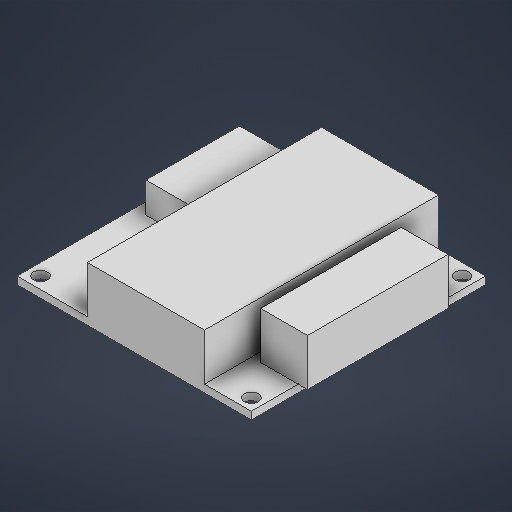
# Autodesk Inventor part: motor_driver
Saved by Autodesk Inventor 2026.2 (Build 302298000, 298)
## iProperties
Created: 2026-03-16
Part Number: motor_driver
Material: Generic
Document SubType Name: Modeling
Designer: User
Density: 1 g/cm^3
Appearance: Default
Author: User
Autodesk Inventor part; units mm, degrees
ref_plane "YZ Plane" through (0, 0, 0) normal (1, 0, 0) x (0, 1, 0)
ref_plane "XZ Plane" through (0, 0, 0) normal (0, 1, 0) x (-1, 0, 0)
ref_plane "XY Plane" through (0, 0, 0) normal (0, 0, 1) x (1, 0, 0)
sketch "Sketch1" plane through (0, 0, 0) normal (0, 1, 0) x (-1, 0, 0)
  line L0 (0, 0) -> (50, 0)
  line L1 (50, 0) -> (50, -50)
  line L2 (50, -50) -> (0, -50)
  line L3 (0, -50) -> (0, 0)
  circle A0 centre (47.5, -2.5) radius 1.5
  circle A1 centre (47.5, -47.5) radius 1.5
  circle A2 centre (2.5, -2.5) radius 1.5
  circle A3 centre (2.5, -47.5) radius 1.5
  dimension "d0" = 50
  dimension "d1" = 50
  dimension "d2" = 3
  dimension "d3" = 3
  dimension "d4" = 3
  dimension "d5" = 3
  dimension "d6" = 2.5
  dimension "d7" = 45
  dimension "d8" = 2.5
  dimension "d9" = 2.5
  dimension "d10" = 2.5
  dimension "d11" = 45
  dimension "d12" = 45
  dimension "d13" = 45
  constraints: 8 end point, 4 centre point, 2 parallel, 1 horizontal, 1 perpendicular
  measures "d0" distance of L1.end L2.end
  measures "d1" distance of L0.end L1.end
  measures "d2" diameter of A0
  measures "d3" diameter of A1
  measures "d4" diameter of A2
  measures "d5" diameter of A3
  measures "d6" distance from line of L1 A0.centre
  measures "d7" distance of A0.centre A2.centre
  measures "d8" distance from line of L0 A0.centre
  measures "d9" distance from line of L1 A1.centre
  measures "d10" distance from line of L0 A2.centre
  measures "d11" distance of A0.centre A1.centre
  measures "d12" distance of A3.centre A1.centre
  measures "d13" distance of A2.centre A3.centre
extrude "Extrusion1" add sketch "Sketch1" along normal blind 1.6
sketch "Sketch2" plane through (0, 1.6, 0) normal (0, 1, 0) x (1, 0, 0)
  line L0 (-10, 0) -> (-35, 0)
  line L1 (-35, 0) -> (-35, 50)
  line L2 (-35, 50) -> (-10, 50)
  line L3 (-10, 50) -> (-10, 0)
  line L4 (-50, 0) -> (0, 0) projected
  line L5 (0, 0) -> (0, 50) projected
  line L6 (2, 10) -> (-8, 10)
  line L7 (-8, 10) -> (-8, 40)
  line L8 (-8, 40) -> (2, 40)
  line L9 (2, 40) -> (2, 10)
  line L10 (-47.5, 45) -> (-38.5, 45)
  line L11 (-38.5, 45) -> (-38.5, 25)
  line L12 (-38.5, 25) -> (-47.5, 25)
  line L13 (-47.5, 25) -> (-47.5, 45)
  line L14 (-50, 50) -> (-50, 0) projected
  line L15 (0, 50) -> (-50, 50) projected
  point P0 (0, 40)
  point P1 (0, 10)
  dimension "d16" = 25
  dimension "d17" = 50
  dimension "d19" = 10
  dimension "d20" = 10
  dimension "d21" = 30
  dimension "d22" = 10
  dimension "d23" = 2
  dimension "d26" = 9
  dimension "d27" = 20
  dimension "d28" = 2.5
  dimension "d29" = 5
  constraints: 24 end point, 6 parallel, 3 horizontal, 3 perpendicular, 1 collinear
  measures "d16" distance of L1.end L2.end
  measures "d17" distance of L0.end L1.end
  measures "d19" distance between parallel lines of L5 L3
  measures "d20" distance of L7.end L8.end
  measures "d21" distance of L6.end L7.end
  measures "d22" distance between parallel lines of L4 L6
  measures "d23" distance between parallel lines of L3 L7
  measures "d26" distance of L11.end L12.end
  measures "d27" distance of L10.end L11.end
  measures "d28" distance between parallel lines of L14 L13
  measures "d29" distance between parallel lines of L10 L15
extrude "Extrusion2" add sketch "Sketch2" along normal blind 10 contours L0 L1 L2 L3 | L6 L7 L8 L5 | L5 L8 L9 L6
extrude "Extrusion3" add sketch "Sketch2" along normal blind 6.5 contours L10 L11 L12 L13
body "Solid1"
